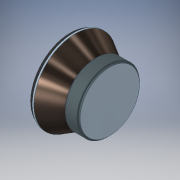
# Autodesk Inventor part: Loudspeaker
Saved by Autodesk Inventor 2018.3 (Build 223284000, 284)
## iProperties
Created: 2018-06-03
Part Number: Loudspeaker
Material: Generisch
Document SubType Name: Modeling
Designer: JochenAlt
Density: 1 g/cm^3
Appearance: Stahlblau
Author: JochenAlt
Autodesk Inventor part; units mm, degrees
ref_plane "YZ Plane" through (0, 0, 0) normal (1, 0, 0) x (0, 1, 0)
ref_plane "XZ Plane" through (0, 0, 0) normal (0, 1, 0) x (-1, 0, 0)
ref_plane "XY Plane" through (0, 0, 0) normal (0, 0, 1) x (1, 0, 0)
sketch "Skizze1" plane through (0, 0, 0) normal (0, 1, 0) x (-1, 0, 0)
  line L0 (37.1685, 22.5) -> (37.1685, 24)
  line L1 (37.1685, 24) -> (35.1685, 24)
  line L2 (35.1685, 24) -> (35.1685, 25)
  line L3 (35.1685, 25) -> (34.1685, 25)
  line L4 (34.1685, 25) -> (22.1685, 18.0718)
  line L5 (22.1685, 18.0718) -> (22.1685, 17.0718)
  line L6 (22.1685, 17.0718) -> (21.1685, 17.0718)
  line L7 (21.1685, 17.0718) -> (21.1685, 19)
  line L8 (21.1685, 19) -> (14.1685, 19)
  line L9 (14.1685, 19) -> (14.1685, 18)
  line L10 (14.1685, 18) -> (13.1685, 18)
  line L11 (13.1685, 18) -> (13.1685, 0)
  line L12 (37.1685, 22.5) -> (34.6685, 22.5)
  arc A0 (34.6685, 18.5) -> (34.6685, 22.5) centre (34.6685, 20.5) ccw
  line L13 (34.6685, 18.5) -> (27.4516, 6)
  arc A1 (29.4516, 0) -> (27.4516, 6) centre (19.4516, 0) ccw
  line L14 (0, -5) -> (0, 30) construction
  line L15 (-7.4337, 0) -> (44.6022, 0) construction
  line L16 (34.6685, 22.5) -> (34.6685, 18.5) construction
  line L17 (29.4516, 0) -> (13.1685, 0)
  point P0 (0, 0)
  dimension "d1" = 2
  dimension "d2" = 30
  dimension "d3" = 6
  dimension "d4" = 22.5
  dimension "d5" = 24
  dimension "d6" = 2
  dimension "d7" = 1
  dimension "d8" = 24
  dimension "d10" = 18
  dimension "d11" = 7
  dimension "d13" = 1
  dimension "d14" = 1
  dimension "d15" = 60
  dimension "d16" = 1
  dimension "d17" = 1
  dimension "d18" = 2
  dimension "d19" = 2.5
  dimension "d20" = 1
  constraints: 32 end point, 8 perpendicular, 4 point on circle, 2 centre point, 2 horizontal, 2 point on line, 2 vertical, 1 line through centre, 1 midpoint, 1 parallel
  measures "d1" radius of A0
  measures "d2" angle of L14 L13
  measures "d3" distance from line of L15 L13.end
  measures "d4" distance between parallel lines of L15 L12
  measures "d5" distance between parallel lines of L15 L1
  measures "d6" distance between parallel lines of L2 L0
  measures "d7" distance of L1.end L2.end
  measures "d8" distance between parallel lines of L11 L0
  measures "d10" distance of L10.end L11.end
  measures "d11" distance of L7.end L8.end
  measures "d13" distance of L9.end L10.end
  measures "d14" distance of L5.end L6.end
  measures "d15" angle of L14 L4
  measures "d16" distance of L8.end L9.end
  measures "d17" distance of L2.end L3.end
  measures "d18" horizontal distance of L17.start L13.end
  measures "d19" distance of L0.start L12.end
  measures "d20" distance of L4.end L5.end
revolve "Umdrehung1" add sketch "Skizze1" angle 360 about axis through (0, 0, 0) along (-1, 0, 0)
